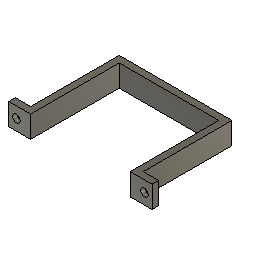
DigitalRegulator_mount_clamp v2 (Autodesk Fusion 360 design; units mm, degrees)
Autodesk Fusion 360 part; units mm, degrees
sketch "Sketch1" plane through (0, 0, 0) normal (0, 0, 1) x (1, 0, 0)
  line L0 (0, 0) -> (7, 0)
  line L1 (7, 0) -> (7, 3)
  line L2 (7, 3) -> (0, 3)
  line L3 (0, 3) -> (0, 0)
  line L4 (7, 0) -> (10, 0)
  line L5 (10, 0) -> (10, 40.5)
  line L6 (10, 40.5) -> (7, 40.5)
  line L7 (7, 40.5) -> (7, 0)
  line L8 (7, 40.5) -> (58.5, 40.5)
  line L9 (58.5, 40.5) -> (58.5, 43.5)
  line L10 (58.5, 43.5) -> (7, 43.5)
  line L11 (7, 43.5) -> (7, 40.5)
  line L12 (58.5, 40.5) -> (55.5, 40.5)
  line L13 (55.5, 40.5) -> (55.5, 0)
  line L14 (55.5, 0) -> (58.5, 0)
  line L15 (58.5, 0) -> (58.5, 40.5)
  line L16 (58.5, 0) -> (65.5, 0)
  line L17 (65.5, 0) -> (65.5, 3)
  line L18 (65.5, 3) -> (58.5, 3)
  line L19 (58.5, 3) -> (58.5, 0)
  dimension "d1" = 7
  dimension "d2" = 3
  dimension "d3" = 3
  dimension "d4" = 40.5
  dimension "d5" = 51.5
  dimension "d6" = 3
  dimension "d7" = 3
  dimension "d8" = 40.5
  dimension "d9" = 7
  dimension "d10" = 3
  constraint horizontal L0
  constraint vertical L1
  constraint horizontal L2
  constraint vertical L3
  constraint coincident L0.start L3.end
  constraint horizontal L4
  constraint vertical L5
  constraint horizontal L6
  constraint vertical L7
  constraint horizontal L8
  constraint vertical L9
  constraint horizontal L10
  constraint vertical L11
  constraint horizontal L12
  constraint vertical L13
  constraint horizontal L14
  constraint vertical L15
  constraint horizontal L16
  constraint vertical L17
  constraint horizontal L18
  constraint vertical L19
  measures "d1" distance of L0.start L0.end
  measures "d2" distance of L0.start L2.end
  measures "d3" distance of L0.end L4.end
  measures "d4" distance of L0.end L6.end
  measures "d5" distance of L6.end L8.end
  measures "d6" distance of L6.end L10.end
  measures "d7" distance of L8.end L12.end
  measures "d8" distance of L8.end L14.end
  measures "d9" distance of L14.end L16.end
  measures "d10" distance of L14.end L18.end
extrude "Extrude1" add sketch "Sketch1" along normal blind 10
sketch "Sketch2" plane through (0, 3, 0) normal (0, 1, 0) x (-1, 0, 0)
  line L0 (-65.5, 0) -> (-58.5, 0)
  line L1 (-58.5, 0) -> (-58.5, 10)
  line L2 (-58.5, 10) -> (-65.5, 10)
  line L3 (-65.5, 10) -> (-65.5, 0)
  point P0 (-62, 5)
  point P1 (-3.5, 5)
hole "Hole1" at (62, 3, 5) at (3.5, 3, 5) direction (0, -1, 0) diameter 3.4 depth 130 tip angle 118 counterbore diameter 5.6 counterbore depth 1
